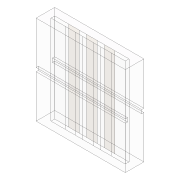
# Autodesk Inventor part: 3_Pin_LED_Verbinder
Saved by Autodesk Inventor 2021.3 (Build 253353000, 353)
## iProperties
Part Number: 3_Pin_LED_Verbinder
Material: PA 6.6
Document SubType Name: Modeling
Designer: SRORF
Mass: 0.337896 g
Surface Area: 6.638 cm^2
Volume: 0.2964 cm^3
Density: 1.14 g/cm^3
Appearance: Lexan (klar)
ROT_Density: 1.0
PDB_Ident_Ver: =<PDB_Ident> <PDB_Version>
ROT_Weight: 0.338 g
ROT_Weight_Num: 0.0003378959999999996
Author: SRORF
Autodesk Inventor part; units mm, degrees
ref_plane "YZ Plane" through (0, 0, 0) normal (1, 0, 0) x (0, 1, 0)
ref_plane "XZ Plane" through (0, 0, 0) normal (0, 1, 0) x (-1, 0, 0)
ref_plane "XY Plane" through (0, 0, 0) normal (0, 0, 1) x (1, 0, 0)
sketch "Skizze2" plane through (0, 0, 0) normal (1, 0, 0) x (0, 1, 0)
  line L0 (1.25, 6) -> (-1.25, 6)
  line L1 (-1.25, 6) -> (-1.25, 0.25)
  line L2 (-1.25, 0.25) -> (-0.95, 0.25)
  line L3 (-0.95, 0.25) -> (-0.95, -0.25)
  line L4 (-0.95, -0.25) -> (-1.25, -0.25)
  line L5 (-1.25, -0.25) -> (-1.25, -6)
  line L6 (-1.25, -6) -> (1.25, -6)
  line L7 (1.25, -6) -> (1.25, -0.25)
  line L8 (1.25, -0.25) -> (0.95, -0.25)
  line L9 (0.95, -0.25) -> (0.95, 0.25)
  line L10 (0.95, 0.25) -> (1.25, 0.25)
  line L11 (1.25, 0.25) -> (1.25, 6)
  line L12 (0.25, 6) -> (0.25, -6) construction
  line L13 (-0.25, -6) -> (-0.25, 6) construction
  point P0 (0, 0)
  point P1 (0.95, 0)
  dimension "d0" = 0.5
  dimension "d1" = 1
  dimension "d2" = 1
  dimension "d3" = 0.5
  dimension "d4" = 0.25
  dimension "d5" = 0.3
  dimension "d6" = 0.3
  dimension "d7" = 6
  dimension "d8" = 6
  constraints: 28 end point, 11 point on line, 9 perpendicular, 1 horizontal, 1 horizontal alignment, 1 midpoint, 1 vertical
  measures "d0" distance between parallel lines of L13 L12
  measures "d1" distance between parallel lines of L7 L12
  measures "d2" distance between parallel lines of L5 L13
  measures "d3" distance of L8.end L9.end
  measures "d4" distance from line of L13 point (0, 0)
  measures "d5" distance between parallel lines of L5 L3
  measures "d6" distance between parallel lines of L7 L9
  measures "d7" distance from line of point (0, 0) L6
  measures "d8" distance from line of point (0, 0) L0
extrude "Extrusion1" add sketch "Skizze2" along normal mid plane 12
sketch "Skizze3" plane through (-6, -1.25, -6) normal (0, 0, -1) x (-1, 0, 0)
  line L0 (-11, 1.5) -> (-1, 1.5)
  line L1 (-1, 1.5) -> (-1, 1)
  line L2 (-1, 1) -> (-11, 1)
  line L3 (-11, 1) -> (-11, 1.5)
  line L4 (0, 2.5) -> (-12, 2.5) projected
  line L5 (0, 2.5) -> (0, 0) projected
  point P0 (-6, 1.25)
  point P1 (-6, 1.5)
  point P2 (-6, 2.5)
  point P3 (-1, 1.25)
  point P4 (0, 1.25)
  dimension "d11" = 10
  dimension "d12" = 0.5
  constraints: 8 end point, 3 midpoint, 2 parallel, 1 horizontal, 1 horizontal alignment, 1 perpendicular, 1 vertical alignment, 2 other
  measures "d11" distance of L0.start L0.end
  measures "d12" distance of L0.end L1.end
extrude "Extrusion2" cut sketch "Skizze3" against normal blind 12
sketch "Skizze4" plane through (-5, -0.25, -6) normal (0, 1, 0) x (1, 0, 0)
  line L0 (-1, -12) -> (11, -12) projected
  line L1 (-1, 0) -> (11, 0) projected
  line L2 (4.3, 0) -> (5.7, 0)
  line L3 (5.7, 0) -> (5.7, -12)
  line L4 (5.7, -12) -> (4.3, -12)
  line L5 (4.3, -12) -> (4.3, 0)
  line L6 (3.3, -12) -> (1.9, -12)
  line L7 (1.9, -12) -> (1.9, 0)
  line L8 (1.9, 0) -> (3.3, 0)
  line L9 (3.3, 0) -> (3.3, -12)
  line L10 (6.7, 0) -> (8.1, 0)
  line L11 (8.1, 0) -> (8.1, -12)
  line L12 (8.1, -12) -> (6.7, -12)
  line L13 (6.7, -12) -> (6.7, 0)
  point P0 (5, -6)
  point P1 (5, -12)
  point P2 (5, -12)
  dimension "d15" = 1.4
  dimension "d16" = 1
  dimension "d17" = 1
  constraints: 24 end point, 6 parallel, 6 point on line, 3 horizontal, 3 perpendicular, 2 collinear, 2 midpoint, 1 coincident
  measures "d15" distance between parallel lines of L3 L5
  measures "d16" distance between parallel lines of L5 L9
  measures "d17" distance between parallel lines of L3 L13
split_face "Trennen1"
split_face "Trennen2"
split_face "Trennen3"
equation "\"d2\" = d1"
equation "\"d4\" = 0.5 * d0"
equation "\"d6\" = d5"
equation "\"d8\" = d7"
equation "\"d17\" = d16"
